Garage Door  Reed Mount (Autodesk Fusion 360 design; units mm, degrees)
Autodesk Fusion 360 part; units mm, degrees
sketch "Sketch1" plane through (0, 0, 0) normal (0, 1, 0) x (1, 0, 0)
  line L0 (0, 0) -> (54, 0)
  line L1 (54, 0) -> (54, -1)
  line L2 (54, -1) -> (0, -1)
  line L3 (0, -1) -> (0, 0)
  line L4 (0, -1) -> (54, -1)
  line L5 (54, -1) -> (54, -6)
  line L6 (54, -6) -> (0, -6)
  line L7 (0, -6) -> (0, -1)
  arc A0 (0, -1) -> (54, -1) centre (27, 69.4) ccw
  dimension "d1" = 54
  dimension "d2" = 1
  dimension "d3" = 5
  constraint horizontal L0
  constraint vertical L1
  constraint horizontal L2
  constraint vertical L3
  constraint coincident L0.start L3.end
  constraint horizontal L4
  constraint vertical L5
  constraint horizontal L6
  constraint vertical L7
  measures "d1" distance of L0.start L0.end
  measures "d2" distance of L0.start L2.end
  measures "d3" distance of L2.end L6.end
extrude "Extrude1" add sketch "Sketch1" along normal blind 15 contours L0 L1 L2 L3 L4 | L2 L4 A0
